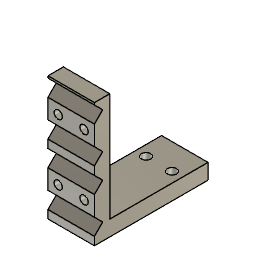
angle v1 (Autodesk Fusion 360 design; units mm, degrees)
Autodesk Fusion 360 part; units mm, degrees
note: some values were not read from the file. Set by a fixed rule: which sketch regions a step uses.
sketch "スケッチ1" plane through (0, 0, 0) normal (0, 0, 1) x (1, 0, 0)
  line L0 (0, 0) -> (-45, 0)
  line L1 (-45, 0) -> (-45, -110)
  line L2 (-45, -110) -> (0, -110)
  line L3 (0, -110) -> (0, 0)
  circle A0 centre (-35, -25) radius 4.5
  circle A1 centre (-10, -25) radius 4.5
  dimension "d1" = 45
  dimension "d2" = 110
  dimension "d3" = 9
  dimension "d4" = 9
  dimension "d5" = 25
  dimension "d6" = 10
  dimension "d7" = 25
  constraint horizontal L0
  constraint vertical L1
  constraint horizontal L2
  constraint vertical L3
  constraint coincident L0.start L3.end
  constraint horizontal A0.centre A1.centre
  measures "d1" distance of L0.start L0.end
  measures "d2" distance of L0.start L2.end
  measures "d3" diameter of A0
  measures "d4" diameter of A1
  measures "d5" distance of A0.centre A1.centre
  measures "d6" distance of L1 A0.centre
  measures "d7" distance of L0 A0.centre
extrude "押し出し1" add sketch "スケッチ1" against normal blind 15 contours L0 L1 L2 L3 | A0 | A1
extrude "押し出し2" cut sketch "スケッチ1" against normal blind 15 contours A0 | A1
sketch "スケッチ2" plane through (0, 0, 0) normal (0, 0, 1) x (1, 0, 0)
  line L0 (0, -95) -> (-45, -95)
  line L1 (-45, -95) -> (-45, -110)
  line L2 (-45, -110) -> (0, -110)
  line L3 (0, -110) -> (0, -95)
  line L4 (0, -110) -> (0, 0)
  point P0 (-45, -110)
  dimension "d12" = 15
  constraint horizontal L0
  constraint vertical L1
  constraint horizontal L2
  constraint vertical L3
  constraint coincident P0 L1.end
  constraint coincident L0.start L4
  measures "d12" distance of L0.start L2.end
extrude "押し出し3" add sketch "スケッチ2" along normal blind 105
sketch "スケッチ3" plane through (0, 0, 0) normal (1, 0, 0) x (0, 1, 0)
  line L0 (-110, 105) -> (-110, -15)
  line L1 (-110, -15) -> (0, -15)
  line L2 (0, -15) -> (0, 0)
  line L3 (0, 0) -> (-95, 0)
  line L4 (-95, 0) -> (-95, 105)
  line L5 (-95, 105) -> (-110, 105)
  line L6 (-110, 95) -> (-102, 95)
  line L7 (-102, 95) -> (-110, 103)
  line L8 (-102, 95) -> (-110, 87)
  circle A0 centre (-117.5091, 95.717) radius 11
  line L9 (-146.8307, 84.717) -> (-108.4644, 84.717)
  line L10 (-108.4644, 84.717) -> (-108.4644, 71.717)
  line L11 (-108.4644, 71.717) -> (-146.8307, 71.717)
  line L12 (-146.8307, 71.717) -> (-146.8307, 84.717)
  circle A1 centre (-117.5091, 60.717) radius 11
  line L13 (-110, 60) -> (-102, 60)
  line L14 (-102, 60) -> (-110, 68)
  line L15 (-102, 60) -> (-110, 52)
  circle A2 centre (-117.5091, 60.717) radius 13
  circle A3 centre (-117.5091, 36.717) radius 11
  line L16 (-102, 36) -> (-110, 28)
  line L17 (-102, 36) -> (-110, 44)
  line L18 (-102, 1) -> (-110, 9)
  line L19 (-102, 1) -> (-110, -7)
  circle A4 centre (-117.5091, 1.717) radius 13
  circle A5 centre (-113.2021, 95.093) radius 7.5
  circle A6 centre (-113.2568, 60.0071) radius 7.5
  dimension "d15" = 8
  dimension "d16" = 45
  dimension "d17" = 22
  dimension "d18" = 13
  dimension "d19" = 38.3662
  dimension "d20" = 22
  dimension "d21" = 8
  dimension "d22" = 45
  dimension "d23" = 35
  dimension "d24" = 26
  dimension "d27" = 0
  dimension "d28" = -59
  dimension "d29" = 2
  dimension "d32" = 15
  dimension "d33" = 15
  constraint coincident L0 L6.start
  constraint perpendicular L0 L6
  constraint perpendicular L7 L8
  constraint coincident L0 L7.end
  constraint coincident L0 L8.end
  constraint horizontal L9
  constraint vertical L10
  constraint horizontal L11
  constraint vertical L12
  constraint tangent A0 L9
  constraint tangent L11 A1
  constraint vertical A0.centre A1.centre
  constraint coincident L0 L13.start
  constraint perpendicular L0 L13
  constraint coincident L0 L14.end
  constraint coincident L0 L15.end
  constraint perpendicular L14 L15
  constraint concentric A1 A2
  measures "d15" distance of L6.start L6.end
  measures "d16" angle of L6 L7
  measures "d17" diameter of A0
  measures "d18" distance of L9.start L11.end
  measures "d19" distance of L10.end L11.end
  measures "d20" diameter of A1
  measures "d21" distance of L13.start L13.end
  measures "d22" angle of L13 L14
  measures "d23" distance of L6.end L13.end
  measures "d24" diameter of A2
  measures "d29" distance of L0.start L7.end
  measures "d32" diameter of A5
  measures "d33" diameter of A6
extrude "押し出し4" cut sketch "スケッチ3" against normal blind 50 contours L0 L18 L19 A4 | L18 L19 A4 | L0 A3 L16 L17 | L0 A3 L17 | L0 A1 L13 L15 A2 A6 | L13 L15 A2 | L0 A1 A6 | L13 L14 A2 | A1 L13 L14 A2 A6 | L0 A1 L14 A6 | L0 A1 L13 A6 | A1 L13 A6 | A1 L13 A6 | L0 A1 L13 A6 | L0 L6 L8 A0 A5 | L0 A0 A5 | L0 L7 A0 A5 | L6 L7 A0 A5 | L0 L6 A0 A5 | L6 A0 A5 | L0 L6 A0 A5 | L6 A0 A5 picked at (-109.6585, 34.1515) picked at (-109.8639, 53.0034) picked at (-109.8537, 88.034)
sketch "スケッチ4" plane through (0, -110, 0) normal (0, -1, 0) x (1, 0, 0)
  line L0 (-45, 68) -> (0, 68)
  line L1 (0, 68) -> (0, 87)
  line L2 (0, 87) -> (-45, 87)
  line L3 (-45, 87) -> (-45, 68)
  circle A0 centre (-35, 77.5) radius 4
  circle A1 centre (-10, 77.5) radius 4
  line L4 (-22.5, 77.5) -> (-22.5, 71.9777)
  line L5 (-45, 105) -> (0, 105)
  circle A2 centre (-35, 18.5) radius 4
  circle A3 centre (-10, 18.5) radius 4
  dimension "d34" = 8
  dimension "d35" = 8
  dimension "d36" = 25
  dimension "d37" = 12.5
  dimension "d38" = 45
  dimension "d39" = 27.5
  dimension "d42" = 0
  dimension "d43" = -59
  constraint vertical L4
  constraint horizontal A0.centre A1.centre
  measures "d34" diameter of A0
  measures "d35" diameter of A1
  measures "d36" distance of A0.centre A1.centre
  measures "d37" distance of A0.centre L4
  measures "d39" distance of A0.centre L5
extrude "押し出し5" cut sketch "スケッチ4" against normal blind 15 contours A0 | A1 | A2 | A3
equation "d13 = 120 mm - 15 mm"
equation "d37 = ( 25 / 2 ) * 1 mm"
